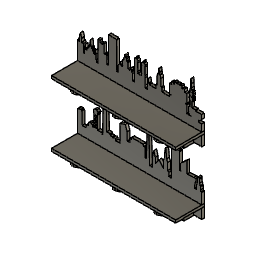
city-skyline-shelf (Autodesk Fusion 360 design; units mm, degrees)
Autodesk Fusion 360 part; units mm, degrees
(part 1 of 2)
sketch "Sketch1" plane through (0, 0, 0) normal (0, 1, 0) x (1, 0, 0) in component "tampere-background"
  line L0 (148.1857, -249.9146) -> (148.1857, -229.9217)
  line L1 (148.1857, -229.9217) -> (137.1896, -228.9221)
  line L2 (137.1896, -228.9221) -> (135.1904, -222.1945)
  line L3 (135.1904, -222.1945) -> (125.1939, -220.9248)
  line L4 (125.1939, -220.9248) -> (125.1939, -214.9267)
  line L5 (125.1939, -214.9267) -> (130.1924, -204.9302)
  line L6 (130.1924, -204.9302) -> (141.1885, -202.931)
  line L7 (141.1885, -202.931) -> (141.1885, -196.9329)
  line L8 (141.1885, -196.9329) -> (135.1904, -195.9333)
  line L9 (135.1904, -195.9333) -> (135.1904, -189.9352)
  line L10 (135.1904, -189.9352) -> (141.1885, -189.9352)
  line L11 (141.1885, -189.9352) -> (139.1893, -62.9787)
  spline S0 degree 3 poles (139.1893, -62.9787) (136.9773, -62.7994) (134.7652, -62.9787) (132.5486, -62.9787) knots 0 0 0 0 1 1 1 1
  line L12 (132.5486, -62.9787) -> (130.1919, -69.9764)
  line L13 (130.1919, -69.9764) -> (110.1989, -69.9764)
  line L14 (110.1989, -69.9764) -> (110.1989, -144.9508)
  line L15 (110.1989, -144.9508) -> (112.1981, -144.9508)
  line L16 (112.1981, -144.9508) -> (112.1981, -154.9473)
  line L17 (112.1981, -154.9473) -> (115.1974, -154.9473)
  line L18 (115.1974, -154.9473) -> (105.2004, -164.9438)
  line L19 (105.2004, -164.9438) -> (95.2039, -164.9438)
  line L20 (95.2039, -164.9438) -> (85.2075, -154.9473)
  line L21 (85.2075, -154.9473) -> (88.2062, -154.9473)
  line L22 (88.2062, -154.9473) -> (88.2062, -144.9508)
  line L23 (88.2062, -144.9508) -> (90.206, -144.9508)
  line L24 (90.206, -144.9508) -> (90.206, -73.9748)
  line L25 (90.206, -73.9748) -> (82.2087, -73.9748)
  line L26 (82.2087, -73.9748) -> (82.2087, -79.9729)
  line L27 (82.2087, -79.9729) -> (84.2079, -79.9729)
  line L28 (84.2079, -79.9729) -> (75.3474, -86.9706)
  line L29 (75.3474, -86.9706) -> (67.3501, -86.9706)
  line L30 (67.3501, -86.9706) -> (58.2168, -79.9729)
  line L31 (58.2168, -79.9729) -> (60.216, -79.9729)
  spline S1 degree 3 poles (60.216, -79.9729) (60.278, -75.6202) (60.3198, -71.3279) (60.216, -66.9771) knots 0 0 0 0 1 1 1 1
  line L32 (60.216, -66.9771) -> (50.2195, -66.9771)
  line L33 (50.2195, -66.9771) -> (45.221, -49.9829)
  line L34 (45.221, -49.9829) -> (25.2281, -49.9829)
  line L35 (25.2281, -49.9829) -> (25.2281, -119.9593)
  line L36 (25.2281, -119.9593) -> (18.2304, -119.9593)
  line L37 (18.2304, -119.9593) -> (18.2304, -124.1964)
  line L38 (18.2304, -124.1964) -> (7.2343, -124.1964)
  line L39 (7.2343, -124.1964) -> (7.2343, -119.9593)
  line L40 (7.2343, -119.9593) -> (0, -119.9593)
  line L41 (0, -119.9593) -> (0, 0)
  line L42 (0, 0) -> (345.1186, 0)
  line L43 (345.1186, 0) -> (690, 0)
  line L44 (690, 0) -> (690, -59.9799)
  line L45 (690, -59.9799) -> (684.0024, -59.9799)
  line L46 (684.0024, -59.9799) -> (684.0024, -69.9764)
  line L47 (684.0024, -69.9764) -> (682.8396, -84.9714)
  line L48 (682.8396, -84.9714) -> (681.0031, -87.9702)
  line L49 (681.0031, -87.9702) -> (678.0043, -98.9662)
  spline S2 degree 3 poles (678.0043, -98.9662) (677.0317, -105.2546) (676.0051, -113.2492) (676.0051, -116.2797) knots 0 0 0 0 1 1 1 1
  line L50 (676.0051, -116.2797) -> (676.0051, -122.2194)
  line L51 (676.0051, -122.2194) -> (672.0062, -128.2175)
  line L52 (672.0062, -128.2175) -> (667.855, -122.2194)
  line L53 (667.855, -122.2194) -> (667.8446, -116.2218)
  spline S3 degree 3 poles (667.8446, -116.2218) (667.8446, -110.2239) (667.0083, -102.9649) (666.0087, -98.9663) knots 0 0 0 0 1 1 1 1
  spline S4 degree 3 poles (666.0087, -98.9663) (665.5521, -97.1399) (664.009, -91.3596) (663.0094, -87.9702) knots 0 0 0 0 1 1 1 1
  line L54 (663.0094, -87.9702) -> (661.0102, -84.9714)
  line L55 (661.0102, -84.9714) -> (660.0044, -69.9764)
  line L56 (660.0044, -69.9764) -> (659.8473, -59.98)
  line L57 (659.8473, -59.98) -> (648.0149, -59.98)
  line L58 (648.0149, -59.98) -> (654.0022, -89.4967)
  spline S5 degree 2 poles (654.0022, -89.4967) (662.7338, -109.7693) (655.0121, -109.9624) knots 0 0 0 1 1 1
  line L59 (655.0121, -109.9624) -> (645.0156, -109.9624)
  line L60 (645.0156, -109.9624) -> (608.0285, -107.4615)
  line L61 (608.0285, -107.4615) -> (608.0285, -173.439)
  line L62 (608.0285, -173.439) -> (573.0405, -143.4491)
  line L63 (573.0405, -143.4491) -> (573.0405, -105.4623)
  line L64 (573.0405, -105.4623) -> (567.1684, -104.9644)
  line L65 (567.1684, -104.9644) -> (567.1684, -194.8345)
  line L66 (567.1684, -194.8345) -> (564.911, -196.7082)
  line L67 (564.911, -196.7082) -> (562.6535, -198.5813)
  line L68 (562.6535, -198.5813) -> (552.3032, -199.5303)
  line L69 (552.3032, -199.5303) -> (541.9528, -200.4788)
  line L70 (541.9528, -200.4788) -> (540.9429, -202.0977)
  line L71 (540.9429, -202.0977) -> (539.933, -203.7167)
  line L72 (539.933, -203.7167) -> (531.8355, -204.2168)
  line L73 (531.8355, -204.2168) -> (523.7385, -204.7168)
  line L74 (523.7385, -204.7168) -> (521.8984, -203.5494)
  line L75 (521.8984, -203.5494) -> (520.0584, -202.3824)
  line L76 (520.0584, -202.3824) -> (520.0584, -110.2563)
  line L77 (520.0584, -110.2563) -> (520.0584, -44.9849)
  line L78 (520.0584, -44.9849) -> (507.0631, -44.9849)
  line L79 (507.0631, -44.9849) -> (507.0631, -64.9779)
  line L80 (507.0631, -64.9779) -> (500.0654, -70.0678)
  line L81 (500.0654, -70.0678) -> (500.0654, -109.9623)
  spline S6 degree 3 poles (500.0654, -109.9623) (499.0397, -115.1717) (497.1361, -120.0402) (495.2121, -124.9573) knots 0 0 0 0 1 1 1 1
  line L82 (495.2121, -124.9573) -> (490.0689, -172.941)
  line L83 (490.0689, -172.941) -> (487.0701, -172.941)
  spline S7 degree 3 poles (487.0701, -172.941) (485.5899, -159.6869) (482.4701, -138.3214) (482.0716, -124.9573) knots 0 0 0 0 1 1 1 1
  spline S8 degree 3 poles (482.0716, -124.9573) (479.9709, -120.0963) (478.5362, -115.0454) (477.1124, -109.9623) knots 0 0 0 0 1 1 1 1
  line L84 (477.1124, -109.9623) -> (477.1124, -70.5457)
  line L85 (477.1124, -70.5457) -> (453.0818, -99.9658)
  line L86 (453.0818, -99.9658) -> (432.2829, -70.9873)
  line L87 (432.2829, -70.9873) -> (431.367, -99.9658)
  line L88 (431.367, -99.9658) -> (424.1157, -129.0399)
  line L89 (424.1157, -129.0399) -> (417.1263, -99.9658)
  spline S9 degree 3 poles (417.1263, -99.9658) (416.743, -92.2664) (416.0777, -52.6248) (415.0945, -44.9849) knots 0 0 0 0 1 1 1 1
  line L90 (415.0945, -44.9849) -> (401.0991, -44.9849)
  line L91 (401.0991, -44.9849) -> (396.1011, -189.9352)
  line L92 (396.1011, -189.9352) -> (386.1046, -189.9352)
  line L93 (386.1046, -189.9352) -> (381.1061, -69.9764)
  line L94 (381.1061, -69.9764) -> (375.108, -69.9764)
  line L95 (375.108, -69.9764) -> (375.108, -119.9593)
  line L96 (375.108, -119.9593) -> (367.0699, -119.9593)
  line L97 (367.0699, -119.9593) -> (364.1119, -129.9558)
  line L98 (364.1119, -129.9558) -> (301.1337, -129.9558)
  line L99 (301.1337, -129.9558) -> (298.1344, -119.9593)
  line L100 (298.1344, -119.9593) -> (290.1371, -119.9593)
  line L101 (290.1371, -119.9593) -> (290.1371, -99.9658)
  line L102 (290.1371, -99.9658) -> (275.1422, -99.9658)
  line L103 (275.1422, -99.9658) -> (275.1422, -144.9508)
  line L104 (275.1422, -144.9508) -> (265.1457, -174.9402)
  line L105 (265.1457, -174.9402) -> (235.1562, -164.9437)
  line L106 (235.1562, -164.9437) -> (235.398, -104.9643)
  line L107 (235.398, -104.9643) -> (235.1562, -69.9764)
  line L108 (235.1562, -69.9764) -> (210.1648, -69.9764)
  line L109 (210.1648, -69.9764) -> (210.1648, -80.0297)
  line L110 (210.1648, -80.0297) -> (198.1686, -79.9729)
  line L111 (198.1686, -79.9729) -> (198.1686, -76.9741)
  line L112 (198.1686, -76.9741) -> (192.171, -76.9741)
  line L113 (192.171, -76.9741) -> (192.171, -79.9729)
  line L114 (192.171, -79.9729) -> (180.1748, -80.0297)
  line L115 (180.1748, -80.0297) -> (180.1748, -87.9702)
  line L116 (180.1748, -87.9702) -> (161.479, -87.9702)
  line L117 (161.479, -87.9702) -> (159.1822, -189.9352)
  line L118 (159.1822, -189.9352) -> (165.1798, -189.9352)
  line L119 (165.1798, -189.9352) -> (165.1798, -195.9333)
  line L120 (165.1798, -195.9333) -> (159.1822, -196.9329)
  line L121 (159.1822, -196.9329) -> (159.1822, -202.931)
  line L122 (159.1822, -202.931) -> (170.1783, -204.9302)
  line L123 (170.1783, -204.9302) -> (175.1768, -214.9267)
  line L124 (175.1768, -214.9267) -> (175.1768, -220.9248)
  line L125 (175.1768, -220.9248) -> (165.1798, -222.4162)
  line L126 (165.1798, -222.4162) -> (163.1806, -228.9221)
  line L127 (163.1806, -228.9221) -> (152.1846, -229.9217)
  line L128 (152.1846, -229.9217) -> (152.1846, -249.9146)
  line L129 (152.1846, -249.9146) -> (148.1857, -249.9146)
  spline S10 degree 3 poles (100.203, -136.9959) (102.1721, -136.9959) (104.1414, -136.9018) (104.5464, -136.7143) knots 0 0 0 0 1 1 1 1
  spline S11 degree 3 poles (104.5464, -136.7143) (105.2015, -136.4111) (105.7342, -135.8601) (106.0094, -135.2012) knots 0 0 0 0 1 1 1 1
  spline S12 degree 3 poles (106.0094, -135.2012) (106.3456, -134.3964) (106.3078, -127.3549) (105.9634, -126.6109) knots 0 0 0 0 1 1 1 1
  spline S13 degree 3 poles (105.9634, -126.6109) (105.2904, -125.1573) (103.3727, -124.4944) (101.8736, -125.197) knots 0 0 0 0 1 1 1 1
  spline S14 degree 3 poles (101.8736, -125.197) (101.1385, -125.5415) (94.6738, -132.0446) (94.3945, -132.7206) knots 0 0 0 0 1 1 1 1
  spline S15 degree 3 poles (94.3945, -132.7206) (93.7727, -134.2253) (94.4455, -136.0597) (95.8595, -136.7143) knots 0 0 0 0 1 1 1 1
  spline S16 degree 3 poles (95.8595, -136.7143) (96.2645, -136.9018) (98.2339, -136.9959) (100.203, -136.9959) knots 0 0 0 0 1 1 1 1
  spline S17 degree 3 poles (97.3545, -120.9992) (97.7556, -120.9853) (98.1565, -120.8949) (98.5313, -120.7192) knots 0 0 0 0 1 1 1 1
  spline S18 degree 3 poles (98.5313, -120.7192) (99.2664, -120.3747) (105.7306, -113.8717) (106.0099, -113.1957) knots 0 0 0 0 1 1 1 1
  spline S19 degree 3 poles (106.0099, -113.1957) (106.6317, -111.6909) (105.9588, -109.8566) (104.5449, -109.2019) knots 0 0 0 0 1 1 1 1
  spline S20 degree 3 poles (104.5449, -109.2019) (103.7348, -108.8269) (96.6685, -108.8269) (95.8585, -109.2019) knots 0 0 0 0 1 1 1 1
  spline S21 degree 3 poles (95.8585, -109.2019) (95.2034, -109.5052) (94.6707, -110.0561) (94.3955, -110.715) knots 0 0 0 0 1 1 1 1
  spline S22 degree 3 poles (94.3955, -110.715) (94.0593, -111.5198) (94.097, -118.5614) (94.4415, -119.3053) knots 0 0 0 0 1 1 1 1
  spline S23 degree 3 poles (94.4415, -119.3053) (94.9462, -120.3955) (96.1511, -121.041) (97.3545, -120.9992) knots 0 0 0 0 1 1 1 1
  spline S24 degree 3 poles (100.203, -103.0075) (102.1721, -103.0075) (104.1414, -102.9135) (104.5464, -102.726) knots 0 0 0 0 1 1 1 1
  spline S25 degree 3 poles (104.5464, -102.726) (105.2015, -102.4227) (105.7342, -101.8718) (106.0094, -101.2129) knots 0 0 0 0 1 1 1 1
  spline S26 degree 3 poles (106.0094, -101.2129) (106.3456, -100.4081) (106.3078, -93.3665) (105.9634, -92.6226) knots 0 0 0 0 1 1 1 1
  spline S27 degree 3 poles (105.9634, -92.6226) (105.2904, -91.1689) (103.3727, -90.5061) (101.8736, -91.2087) knots 0 0 0 0 1 1 1 1
  spline S28 degree 3 poles (101.8736, -91.2087) (101.1385, -91.5532) (94.6738, -98.0562) (94.3945, -98.7322) knots 0 0 0 0 1 1 1 1
  spline S29 degree 3 poles (94.3945, -98.7322) (93.7727, -100.237) (94.4455, -102.0713) (95.8595, -102.726) knots 0 0 0 0 1 1 1 1
  spline S30 degree 3 poles (95.8595, -102.726) (96.2645, -102.9135) (98.2339, -103.0075) (100.203, -103.0075) knots 0 0 0 0 1 1 1 1
  spline S31 degree 3 poles (97.3545, -87.0109) (97.7556, -86.997) (98.1565, -86.9065) (98.5313, -86.7309) knots 0 0 0 0 1 1 1 1
  spline S32 degree 3 poles (98.5313, -86.7309) (99.2664, -86.3863) (105.7306, -79.8833) (106.0099, -79.2073) knots 0 0 0 0 1 1 1 1
  spline S33 degree 3 poles (106.0099, -79.2073) (106.6317, -77.7025) (105.9588, -75.8682) (104.5449, -75.2136) knots 0 0 0 0 1 1 1 1
  spline S34 degree 3 poles (104.5449, -75.2136) (103.7348, -74.8385) (96.6685, -74.8385) (95.8585, -75.2136) knots 0 0 0 0 1 1 1 1
  spline S35 degree 3 poles (95.8585, -75.2136) (95.2034, -75.5168) (94.6707, -76.0678) (94.3955, -76.7266) knots 0 0 0 0 1 1 1 1
  spline S36 degree 3 poles (94.3955, -76.7266) (94.0593, -77.5314) (94.097, -84.573) (94.4415, -85.317) knots 0 0 0 0 1 1 1 1
  spline S37 degree 3 poles (94.4415, -85.317) (94.9462, -86.4072) (96.1511, -87.0526) (97.3545, -87.0109) knots 0 0 0 0 1 1 1 1
  line L130 (138, 0) -> (276, 0)
  line L131 (414, 0) -> (552, 0)
  line L132 (0, 0) -> (690, 0)
  line L133 (690, 70) -> (0, 70)
  line L134 (138, 15.1) -> (138, 0)
  line L135 (0, 15.1) -> (0, 70)
  line L136 (276, 0) -> (414, 0)
  line L137 (414, 0) -> (414, 15.1)
  line L138 (276, 15.1) -> (276, 0)
  line L139 (552, 0) -> (552, 15.1)
  line L140 (690, 15.1) -> (690, 70)
  line L141 (337.45, 15.1) -> (337.45, 44.6036)
  line L142 (337.45, 44.6036) -> (352.55, 44.6036)
  line L143 (352.55, 44.6036) -> (352.55, 15.1)
  line L144 (106, 15.1) -> (106, 44.6036)
  line L145 (106, 44.6036) -> (121.1, 44.6036)
  line L146 (121.1, 44.6036) -> (121.1, 15.1)
  line L147 (584, 15.1) -> (584, 44.6036)
  line L148 (584, 44.6036) -> (568.9, 44.6036)
  line L149 (568.9, 44.6036) -> (568.9, 15.1)
  line L150 (121.1, 15.1) -> (138, 15.1)
  line L151 (106, 15.1) -> (0, 15.1)
  line L152 (276, 15.1) -> (337.45, 15.1)
  line L153 (352.55, 15.1) -> (414, 15.1)
  line L154 (552, 15.1) -> (568.9, 15.1)
  line L155 (584, 15.1) -> (690, 15.1)
  dimension "d110" = 70
  dimension "d112" = 15.1
  dimension "d113" = 138
  dimension "d115" = 138
  dimension "d116" = 15.1
  dimension "d117" = 138
  dimension "d118" = 15.1
  dimension "d119" = 138
  dimension "d127" = 15.1
  dimension "d128" = 61.45
  dimension "d129" = 29.5036
  dimension "d130" = 106
  dimension "d131" = 15.1
  dimension "d132" = 29.5036
  dimension "d133" = 106
  dimension "d134" = 29.5036
  dimension "d135" = 15.1
  dimension "d158" = 15.1
  dimension "d159" = 15.1
  dimension "d160" = 15.1
  constraint horizontal L130
  constraint coincident L42 L130.start
  constraint horizontal L131
  constraint coincident L43 L131.start
  constraint horizontal L132
  constraint horizontal L133
  constraint coincident L41.end L42.start
  constraint perpendicular L132 L134
  constraint perpendicular L133 L135
  constraint equal L132 L133
  constraint horizontal L136
  constraint vertical L137
  constraint vertical L138
  constraint coincident L132 L130.end
  constraint coincident L43 L131.end
  constraint perpendicular L43 L139
  constraint perpendicular L133 L140
  constraint vertical L141
  constraint horizontal L142
  constraint vertical L143
  constraint vertical L144
  constraint horizontal L145
  constraint vertical L146
  constraint vertical L147
  constraint horizontal L148
  constraint vertical L149
  constraint horizontal L151
  constraint horizontal L150
  constraint perpendicular L141 L152
  constraint perpendicular L137 L153
  constraint perpendicular L149 L154
  constraint perpendicular L140 L155
  constraint collinear L44 L140
  constraint collinear L41 L135
  measures "d110" distance of L43.end L133.start
  measures "d112" distance of L130.start L134.start
  measures "d113" distance of L134.start L135.start
  measures "d115" distance of L137.end L138.start
  measures "d116" distance of L131.start L137.end
  measures "d117" distance of L134 L138
  measures "d118" distance of L131.end L139.end
  measures "d119" distance of L139.end L140.start
  measures "d127" distance of L141.end L142.end
  measures "d128" distance of L137.end L143
  measures "d129" distance of L141.start L141.end
  measures "d130" distance of L135 L144
  measures "d131" distance of L144.end L145.end
  measures "d132" distance of L146.end L145.end
  measures "d133" distance of L140 L147
  measures "d134" distance of L149.end L148.end
  measures "d135" distance of L147.end L148.end
  measures "d158" distance of L42 L151
  measures "d159" distance of L132 L155
  measures "d160" distance of L42 L152
extrude "Extrude1" add sketch "Sketch1" along normal blind 15 contours L0 L1 L2 L3 L4 L5 L6 L7 L8 L9 L10 L11 S0 L12 L13 L14 L15 L16 L17 L18 L19 L20 L21 L22 L23 L24 L25 L26 L27 L28 L29 L30 L31 S1 L32 L33 L34 L35 L36 L37 L38 L39 L40 L41 L42 L43 L44 L45 L46 L47 L48 L49 S2 L50 L51 L52 L53 S3 S4 L54 L55 L56 L57 L58 S5 L59 L60 L61 L62 L63 L64 L65 L66 L67 L68 L69 L70 L71 L72 L73 L74 L75 L76 L77 L78 L79 L80 L81 S6 L82 L83 S7 S8 L84 L85 L86 L87 L88 L89 S9 L90 L91 L92 L93 L94 L95 L96 L97 L98 L99 L100 L101 L102 L103 L104 L105 L106 L107 L108 L109 L110 L111 L112 L113 L114 L115 L116 L117 L118 L119 L120 L121 L122 L123 L124 L125 L126 L127 L128 L129 L130 L131 L132 L136 | L42 L43 L130 L131 L132 L133 L134 L135 L137 L138 L139 L140 L141 L142 L143 L144 L145 L146 L147 L148 L149 L150 L151 L152 L153 L154 L155 makes body 1 in component "tampere-background"
sketch "Sketch2" plane through (0, 0, 0) normal (0, 0, 1) x (1, 0, 0) in component "shelf"
  line L0 (0, 0) -> (690, 0)
  line L1 (690, 0) -> (690, -145)
  line L2 (690, -145) -> (0, -145)
  line L3 (0, -145) -> (0, 0)
  line L4 (0, 0) -> (138, 0)
  line L5 (138, 0) -> (138, 15)
  line L6 (138, 15) -> (0, 15)
  line L7 (0, 15) -> (0, 0)
  line L8 (552, 0) -> (690, 0)
  line L9 (690, 0) -> (690, 15)
  line L10 (690, 15) -> (552, 15)
  line L11 (552, 15) -> (552, 0)
  line L12 (276, 0) -> (414, 0)
  line L13 (414, 0) -> (414, 15)
  line L14 (414, 15) -> (276, 15)
  line L15 (276, 15) -> (276, 0)
  dimension "d12" = 690
  dimension "d13" = 145
  dimension "d14" = 138
  dimension "d16" = 15
  dimension "d17" = 138
  dimension "d18" = 15
  dimension "d30" = 138
  dimension "d31" = 15
  dimension "d32" = 138
  constraint horizontal L0
  constraint vertical L1
  constraint horizontal L2
  constraint vertical L3
  constraint coincident L0.start L3.end
  constraint horizontal L4
  constraint vertical L5
  constraint horizontal L6
  constraint vertical L7
  constraint coincident L0 L3.end
  constraint horizontal L8
  constraint vertical L9
  constraint horizontal L10
  constraint vertical L11
  constraint coincident L0 L8.start
  constraint coincident L0.start L7
  constraint coincident L0.end L9
  constraint horizontal L12
  constraint vertical L13
  constraint horizontal L14
  constraint vertical L15
  constraint coincident L0 L12.start
  measures "d12" distance of L1.end L2.end
  measures "d13" distance of L0.start L2.end
  measures "d14" distance of L5.end L6.end
  measures "d16" distance of L0.start L6.end
  measures "d17" distance of L9.end L10.end
  measures "d18" distance of L0.end L9.end
  measures "d30" distance of L13.end L14.end
  measures "d31" distance of L12.end L13.end
  measures "d32" distance of L11 L13
extrude "Extrude1'" add sketch "Sketch2" along normal blind 15 separate body makes body 2 in component "shelf"
move_body "Move1" bodies 2 to x (1, 0, 0) y (0, 1, 0) z (0, 0, 1) at (0, 0, -75) in component "shelf"
sketch "Sketch4" plane through (0, 0, -75) normal (0, 0, -1) x (1, 0, 0)
  line L0 (414, -15) -> (414, 0)
  line L1 (414, 0) -> (552, 0)
  line L2 (552, 0) -> (552, -15)
  line L3 (552, -15) -> (690, -15)
  line L4 (690, -15) -> (690, 145)
  line L5 (690, 145) -> (0, 145)
  line L6 (0, 145) -> (0, -15)
  line L7 (0, -15) -> (138, -15)
  line L8 (138, -15) -> (138, 0)
  line L9 (138, 0) -> (276, 0)
  line L10 (276, 0) -> (276, -15)
  line L11 (276, -15) -> (414, -15)
  line L12 (106, -15) -> (121.1, -15)
  line L13 (121.1, -15) -> (121.1, 141.8)
  line L14 (121.1, 141.8) -> (106, 141.8)
  line L15 (106, 141.8) -> (106, -15)
  line L16 (337.45, -15) -> (352.55, -15)
  line L17 (352.55, -15) -> (352.55, 141.8)
  line L18 (352.55, 141.8) -> (337.45, 141.8)
  line L19 (337.45, 141.8) -> (337.45, -15)
  line L20 (568.9, -15) -> (584, -15)
  line L21 (584, -15) -> (584, 141.8)
  line L22 (584, 141.8) -> (568.9, 141.8)
  line L23 (568.9, 141.8) -> (568.9, -15)
  line L24 (121.1, 113.6693) -> (337.45, 113.6693) construction
  line L25 (352.55, 113.6693) -> (568.9, 113.6693) construction
  line L26 (0, 99.2167) -> (690, 99.2167)
  line L27 (690, 99.2167) -> (690, 45.7833)
  line L28 (690, 45.7833) -> (0, 45.7833)
  line L29 (0, 45.7833) -> (0, 99.2167)
  line L30 (690, 72.5) -> (690, 65) construction
  dimension "d43" = 15.1
  dimension "d44" = 156.8
  dimension "d45" = 106
  dimension "d46" = 106
  dimension "d48" = 53.4333
  dimension "d145" = 45.7833
  constraint horizontal L12
  constraint vertical L13
  constraint horizontal L14
  constraint vertical L15
  constraint horizontal L16
  constraint vertical L17
  constraint horizontal L18
  constraint vertical L19
  constraint horizontal L20
  constraint vertical L21
  constraint horizontal L22
  constraint vertical L23
  constraint equal L14 L18
  constraint equal L18 L22
  constraint equal L13 L17
  constraint equal L17 L21
  constraint coincident L13 L24.start
  constraint coincident L19 L24.end
  constraint perpendicular L19 L24
  constraint coincident L17 L25.start
  constraint coincident L23 L25.end
  constraint perpendicular L23 L25
  constraint equal L24 L25
  constraint horizontal L26
  constraint vertical L27
  constraint horizontal L28
  constraint vertical L29
  constraint midpoint L27 L30.start
  constraint midpoint L4 L30.end
  constraint coincident L19 L16.start
  constraint coincident L20.start L23.end
  constraint coincident L12.start L15.end
  constraint coincident L16.start L19.end
  constraint collinear L11 L16
  constraint collinear L3 L20
  constraint collinear L7 L12
  constraint collinear L6 L29
  constraint collinear L4 L27
  measures "d43" distance of L17.end L18.end
  measures "d44" distance of L16.end L17.end
  measures "d45" distance of origin L15
  measures "d46" distance of L3.end L21
  measures "d48" distance of L26.end L27.end
  measures "d145" distance of L1 L28
extrude "Extrude2" cut sketch "Sketch4" against normal blind 1.875 contours L11 L16 L17 L19 L28 | L17 L19 L26 L28 | L17 L23 L26 L28 | L13 L19 L26 L28 | L17 L18 L19 L26 | L3 L20 L21 L23 L28 | L21 L23 L26 L28 | L13 L15 L26 L28 | L7 L12 L13 L15 L28 | L21 L22 L23 L26 | L4 L21 L26 L27 L28 | L13 L14 L15 L26 | L6 L15 L26 L28 L29 bodies 2 in component "shelf"
sketch "Sketch1 (2)" plane through (0, 0, 0) normal (0, 0, 1) x (1, 0, 0) in component "support-bar"
sketch "Sketch2 (2)" plane through (0, 0, 0) normal (0, 0, 1) x (1, 0, 0) in component "support-bar"
  line L0 (0, 0) -> (690, 0)
  line L1 (690, 0) -> (690, -53.3333)
  line L2 (690, -53.3333) -> (0, -53.3333)
  line L3 (0, -53.3333) -> (0, 0)
  dimension "d52" = 690
  dimension "d53" = 53.3333
  constraint horizontal L0
  constraint vertical L1
  constraint horizontal L2
  constraint vertical L3
  constraint coincident L0.start L3.end
  measures "d52" distance of L0.start L0.end
  measures "d53" distance of L0.start L2.end
extrude "Extrude1''" add sketch "Sketch2 (2)" along normal blind 15 separate body makes body 3 in component "support-bar"
move_body "Move1'" bodies 3 to x (1, 0, 0) y (0, 1, 0) z (0, 0, 1) at (0, 0, -90) in component "support-bar"
sketch "Sketch1 (3)" plane through (0, 0, 0) normal (1, 0, 0) x (0, 1, 0) in component "triangle-support"
  line L0 (-15, 0) -> (-150, 0)
  line L1 (-155.4076, -18.4118) -> (-15.4076, -108.4118)
  line L2 (0, -100) -> (0, -56.925)
  arc A0 (-15.4076, -108.4118) -> (0, -100) centre (-10, -100) ccw
  arc A1 (-150, 0) -> (-155.4076, -18.4118) centre (-150, -10) ccw
  line L3 (0, 0) -> (0, -110) construction
  line L4 (0, 0) -> (-160, 0) construction
  line L5 (0, -110) -> (-35, -110) construction
  line L6 (-160, 0) -> (-160, -24.9001) construction
  line L7 (-45, -31.3786) -> (-77.5293, -31.3786)
  line L8 (-80.2331, -40.5845) -> (-47.7038, -61.4962)
  line L9 (-40, -57.2903) -> (-40, -36.3786)
  arc A2 (-47.7038, -61.4962) -> (-40, -57.2903) centre (-45, -57.2903) ccw
  arc A3 (-40, -36.3786) -> (-45, -31.3786) centre (-45, -36.3786) ccw
  arc A4 (-77.5293, -31.3786) -> (-80.2331, -40.5845) centre (-77.5293, -36.3786) ccw
  line L10 (-60.7833, 0) -> (-114.2167, 0)
  line L11 (-114.2167, 0) -> (-114.2167, -15)
  line L12 (-114.2167, -15) -> (-60.7833, -15)
  line L13 (-60.7833, -15) -> (-60.7833, 0)
  line L14 (0, -56.925) -> (-15, -56.925)
  line L15 (-15, -56.925) -> (-15, 0)
  line L16 (-15, 0) -> (0, 0)
  line L17 (0, 0) -> (0, -31.3786)
  line L18 (0, -31.3786) -> (-15, -31.3786)
  line L19 (-66.4844, -49.4229) -> (-78.3811, -67.9288) construction
  dimension "d60" = 10
  dimension "d63" = 110
  dimension "d64" = 160
  dimension "d65" = 5
  dimension "d66" = 5
  dimension "d67" = 40
  dimension "d68" = 31.3786
  dimension "d71" = 53.4333
  dimension "d72" = 15
  dimension "d124" = 15
  dimension "d125" = 56.925
  dimension "d126" = 15
  dimension "d136" = 45.7833
  dimension "d186" = 22
  constraint horizontal L0
  constraint perpendicular L0 L2
  constraint tangent L2 A0
  constraint tangent L1 A0
  constraint tangent L1 A1
  constraint tangent L0 A1
  constraint equal A0 A1
  constraint coincident L3.start L4.start
  constraint perpendicular L0 L3
  constraint collinear L2 L3
  constraint perpendicular L3 L4
  constraint collinear L0 L4
  constraint horizontal L5
  constraint tangent A0 L5
  constraint coincident L3.end L5.start
  constraint vertical L6
  constraint tangent A1 L6
  constraint coincident L4.end L6.start
  constraint parallel L4 L7
  constraint perpendicular L7 L9
  constraint tangent L8 A2
  constraint tangent L9 A2
  constraint tangent L9 A3
  constraint tangent L7 A3
  constraint equal A2 A3
  constraint tangent L7 A4
  constraint tangent L8 A4
  constraint horizontal L10
  constraint vertical L11
  constraint horizontal L12
  constraint vertical L13
  constraint coincident L4 L10.start
  constraint coincident L0 L10.start
  constraint horizontal L14
  constraint vertical L15
  constraint coincident L2 L14.start
  constraint coincident L3 L2.end
  constraint coincident L4 L0.start
  constraint coincident L2.end L14.start
  constraint coincident L0.start L15.end
  constraint horizontal L16
  constraint vertical L17
  constraint horizontal L18
  constraint collinear L7 L18
  constraint parallel L1 L8
  constraint coincident L8 L19.start
  constraint coincident L1 L19.end
  constraint perpendicular L1 L19
  constraint coincident L15 L18.end
  measures "d60" radius of A0
  measures "d63" distance of L3.start L3.end
  measures "d64" distance of L3.start L4.end
  measures "d65" radius of A2
  measures "d66" radius of A4
  measures "d67" distance of L2 L9
  measures "d68" distance of L0 L7
  measures "d71" distance of L11.end L12.end
  measures "d72" distance of L10.end L11.end
  measures "d124" distance of L2.end L14.end
  measures "d125" distance of L0.start L14.end
  measures "d126" distance of L0.start L3.start
  measures "d136" distance of L13 L15
  measures "d186" distance of L19.start L19.end
extrude "Extrude1'''" add sketch "Sketch1 (3)" along normal blind 15 separate body contours L0 L1 L2 A0 A1 L11 L12 L13 L14 L15 | L15 L16 L17 L18 makes body 4 in component "triangle-support"
move_body "Move1''" bodies 4 to x (1, 0, 0) y (0, 1, 0) z (0, 0, 1) at (0, 0, -50) in component "triangle-support"
sketch "Sketch1 (4)" plane through (0, 0, 0) normal (0, 1, 0) x (1, 0, 0) in component "munich-background"
  line L0 (629, -226.9948) -> (628, -204.9948)
  line L1 (628, -204.9948) -> (627, -184.9948)
  line L2 (627, -184.9948) -> (625, -174.9948)
  line L3 (625, -174.9948) -> (625, -169.9948)
  line L4 (625, -169.9948) -> (623, -169.9948)
  spline S0 degree 3 poles (623, -169.9948) (622.0426, -169.9666) (621, -168.9522) (621, -167.9948) knots 0 0 0 0 1 1 1 1
  spline S1 degree 3 poles (621, -167.9948) (621.0282, -166.9529) (622.0426, -166.0229) (623, -165.9948) knots 0 0 0 0 1 1 1 1
  line L5 (623, -165.9948) -> (625, -165.9948)
  line L6 (625, -165.9948) -> (625, -159.9948)
  line L7 (625, -159.9948) -> (619, -157.9948)
  line L8 (619, -157.9948) -> (619, -147.9948)
  line L9 (619, -147.9948) -> (625, -145.9948)
  line L10 (625, -145.9948) -> (625, -139.9948)
  line L11 (625, -139.9948) -> (619, -139.9948)
  line L12 (619, -139.9948) -> (619, -137.9948)
  spline S2 degree 2 poles (619, -137.9948) (621, -137.9948) (621, -134.9948) knots 0 0 0 1 1 1
  spline S3 degree 2 poles (621, -134.9948) (621, -131.9948) (619, -131.9948) knots 0 0 0 1 1 1
  line L13 (619, -131.9948) -> (619, -129.9948)
  spline S4 degree 2 poles (619, -129.9948) (621, -129.9948) (621, -126.9948) knots 0 0 0 1 1 1
  spline S5 degree 2 poles (621, -126.9948) (621, -123.9948) (619, -123.9948) knots 0 0 0 1 1 1
  line L14 (619, -123.9948) -> (619, -121.9948)
  line L15 (619, -121.9948) -> (625, -121.9948)
  line L16 (625, -121.9948) -> (624, -89.9948)
  line L17 (624, -89.9948) -> (617, -89.9948)
  line L18 (617, -89.9948) -> (617, -61.9948)
  spline S6 degree 3 poles (617, -61.9948) (617, -55.9948) (623, -47.9948) (630, -47.9948) knots 0 0 0 0 1 1 1 1
  line L19 (630, -47.9948) -> (607.0867, -47.9948)
  line L20 (607.0867, -47.9948) -> (607.0867, -89.9948)
  line L21 (607.0867, -89.9948) -> (599, -93.9948)
  line L22 (599, -93.9948) -> (607.1813, -97.9948)
  line L23 (607.1813, -97.9948) -> (607, -144.9948)
  line L24 (607, -144.9948) -> (595, -144.9948)
  line L25 (595, -144.9948) -> (594.9041, -159.9948)
  line L26 (594.9041, -159.9948) -> (587, -159.9948)
  spline S7 degree 2 poles (587, -159.9948) (587, -153.0676) (580, -154.9948) knots 0 0 0 1 1 1
  line L27 (580, -154.9948) -> (580, -166.9948)
  line L28 (580, -166.9948) -> (570, -166.9948)
  line L29 (570, -166.9948) -> (570, -164.9948)
  line L30 (570, -164.9948) -> (564, -164.9948)
  line L31 (564, -164.9948) -> (564, -166.9948)
  line L32 (564, -166.9948) -> (553, -166.9948)
  line L33 (553, -166.9948) -> (553, -164.9948)
  line L34 (553, -164.9948) -> (547, -164.9948)
  line L35 (547, -164.9948) -> (547, -166.9948)
  line L36 (547, -166.9948) -> (537, -166.9948)
  line L37 (537, -166.9948) -> (537, -154.9948)
  spline S8 degree 2 poles (537, -154.9948) (529.9203, -153.1452) (530, -159.9948) knots 0 0 0 1 1 1
  line L38 (530, -159.9948) -> (522, -159.9948)
  line L39 (522, -159.9948) -> (521.991, -145.2144)
  line L40 (521.991, -145.2144) -> (510, -145.2144)
  line L41 (510, -145.2144) -> (510, -97.9948)
  line L42 (510, -97.9948) -> (518, -93.9948)
  line L43 (518, -93.9948) -> (510, -89.9948)
  line L44 (510, -89.9948) -> (510, -82.9948)
  line L45 (510, -82.9948) -> (469, -82.9948)
  line L46 (469, -82.9948) -> (469, -102.9948)
  line L47 (469, -102.9948) -> (463, -102.9948)
  line L48 (463, -102.9948) -> (463, -144.9948)
  line L49 (463, -144.9948) -> (459, -159.9948)
  line L50 (459, -159.9948) -> (456, -159.9948)
  line L51 (456, -159.9948) -> (456, -169.9948)
  line L52 (456, -169.9948) -> (454, -169.9948)
  line L53 (454, -169.9948) -> (453, -187.9948)
  spline S9 degree 2 poles (453, -187.9948) (452.115, -192.5346) (451, -187.9948) knots 0 0 0 1 1 1
  line L54 (451, -187.9948) -> (450, -169.9948)
  line L55 (450, -169.9948) -> (448, -169.9948)
  line L56 (448, -169.9948) -> (448, -159.9948)
  line L57 (448, -159.9948) -> (445, -159.9948)
  line L58 (445, -159.9948) -> (441, -144.9948)
  line L59 (441, -144.9948) -> (441, -102.9948)
  line L60 (441, -102.9948) -> (435, -102.9948)
  line L61 (435, -102.9948) -> (435, -82.9948)
  line L62 (435, -82.9948) -> (398, -82.9948)
  line L63 (398, -82.9948) -> (398, -85.9948)
  spline S10 degree 2 poles (398, -85.9948) (396, -86.1933) (396, -89.9948) knots 0 0 0 1 1 1
  line L64 (396, -89.9948) -> (395, -89.9948)
  line L65 (395, -89.9948) -> (393, -109.9948)
  spline S11 degree 2 poles (393, -109.9948) (392.5376, -112.3045) (392, -109.9948) knots 0 0 0 1 1 1
  line L66 (392, -109.9948) -> (390, -89.9948)
  line L67 (390, -89.9948) -> (389, -89.9948)
  spline S12 degree 2 poles (389, -89.9948) (388.9155, -85.9399) (387, -85.9948) knots 0 0 0 1 1 1
  line L68 (387, -85.9948) -> (387, -77.9948)
  line L69 (387, -77.9948) -> (386, -77.9948)
  spline S13 degree 2 poles (386, -77.9948) (385, -77.9804) (385, -76.9948) knots 0 0 0 1 1 1
  line L70 (385, -76.9948) -> (385, -74.9948)
  spline S14 degree 2 poles (385, -74.9948) (385.0563, -73.9529) (385.9771, -73.9948) knots 0 0 0 1 1 1
  line L71 (385.9771, -73.9948) -> (387, -73.9948)
  line L72 (387, -73.9948) -> (387, -66.9948)
  line L73 (387, -66.9948) -> (386, -66.9948)
  spline S15 degree 2 poles (386, -66.9948) (385.0282, -66.9804) (385, -65.9948) knots 0 0 0 1 1 1
  line L74 (385, -65.9948) -> (385, -62.9948)
  spline S16 degree 2 poles (385, -62.9948) (385.0282, -62.0092) (385.9208, -61.9948) knots 0 0 0 1 1 1
  line L75 (385.9208, -61.9948) -> (387, -61.9948)
  line L76 (387, -61.9948) -> (387, -55.0799)
  line L77 (387, -55.0799) -> (374.9999, -54.9948)
  line L78 (374.9999, -54.9948) -> (375, -104.9947)
  line L79 (375, -104.9947) -> (375, -114.9948)
  line L80 (375, -114.9948) -> (374, -154.9948)
  line L81 (374, -154.9948) -> (374.9999, -164.8056)
  spline S17 degree 2 poles (374.9999, -164.8056) (375.0125, -172.3049) (370.0002, -172.4175) knots 0 0 0 1 1 1
  line L82 (370.0002, -172.4175) -> (366, -172.9952)
  line L83 (366, -172.9952) -> (365.2558, -179.9948)
  spline S18 degree 2 poles (365.2558, -179.9948) (365.1621, -180.2093) (365.0315, -180.2361) knots 0 0 0 1 1 1
  spline S19 degree 3 poles (365.0315, -180.2361) (364.9532, -180.2522) (364.8619, -180.2007) (364.7696, -179.9948) knots 0 0 0 0 1 1 1 1
  line L84 (364.7696, -179.9948) -> (364.0001, -172.9952)
  line L85 (364.0001, -172.9952) -> (360.0003, -172.4454)
  spline S20 degree 2 poles (360.0003, -172.4454) (354.988, -172.4454) (355.0001, -164.9952) knots 0 0 0 1 1 1
  spline S21 degree 3 poles (355.0001, -164.9952) (354.9567, -160.9839) (356.0148, -158.9586) (356.0001, -154.9948) knots 0 0 0 0 1 1 1 1
  spline S22 degree 3 poles (356.0001, -154.9948) (355.9538, -142.5116) (355.0924, -127.2661) (355, -114.9948) knots 0 0 0 0 1 1 1 1
  spline S23 degree 3 poles (355, -114.9948) (354.9666, -109.6615) (355, -110.328) (355, -104.9947) knots 0 0 0 0 1 1 1 1
  line L86 (355, -104.9947) -> (335.0002, -104.9947)
  line L87 (335.0002, -104.9947) -> (335.0002, -114.9946)
  line L88 (335.0002, -114.9946) -> (333.9998, -154.9947)
  line L89 (333.9998, -154.9947) -> (335.0002, -164.8055)
  spline S24 degree 2 poles (335.0002, -164.8055) (335.0123, -172.3048) (330, -172.4174) knots 0 0 0 1 1 1
  line L90 (330, -172.4174) -> (326.0002, -172.9946)
  line L91 (326.0002, -172.9946) -> (325.2561, -179.9947)
  spline S25 degree 2 poles (325.2561, -179.9947) (325.0157, -180.5438) (324.7693, -179.9947) knots 0 0 0 1 1 1
  line L92 (324.7693, -179.9947) -> (323.9998, -172.9946)
  line L93 (323.9998, -172.9946) -> (320.0001, -172.4453)
  spline S26 degree 2 poles (320.0001, -172.4453) (314.9878, -172.4453) (314.9999, -164.9946) knots 0 0 0 1 1 1
  spline S27 degree 3 poles (314.9999, -164.9946) (314.9565, -160.9833) (316.0145, -158.9586) (315.9998, -154.9947) knots 0 0 0 0 1 1 1 1
  spline S28 degree 3 poles (315.9998, -154.9947) (315.9497, -141.4944) (314.9542, -128.2723) (314.9999, -114.9946) knots 0 0 0 0 1 1 1 1
  spline S29 degree 3 poles (314.9999, -114.9946) (315.068, -95.1907) (315.077, -75.3722) (314.9999, -54.9946) knots 0 0 0 0 1 1 1 1
  line L94 (314.9999, -54.9946) -> (305, -54.9946)
  line L95 (305, -54.9946) -> (305, -89.9945)
  spline S30 degree 3 poles (305, -89.9945) (303.7059, -91.7055) (304.9998, -92.995) (299.9476, -95.003) knots 0 0 0 0 1 1 1 1
  line L96 (299.9476, -95.003) -> (299.9998, -94.995)
  spline S31 degree 2 poles (299.9998, -94.995) (301.2741, -97.4864) (299.9998, -99.9952) knots 0 0 0 1 1 1
  spline S32 degree 2 poles (299.9998, -99.9952) (298.9999, -100.9952) (296.9999, -100.9952) knots 0 0 0 1 1 1
  spline S33 degree 3 poles (296.9999, -100.9952) (296.5852, -100.9952) (295.9435, -108.302) (294.9995, -109.9952) knots 0 0 0 0 1 1 1 1
  spline S34 degree 3 poles (294.9995, -109.9952) (294.3124, -111.2275) (293.6213, -111.1943) (292.9997, -109.9952) knots 0 0 0 0 1 1 1 1
  spline S35 degree 3 poles (292.9997, -109.9952) (292.7185, -109.4528) (291.5277, -101.0168) (290.9998, -100.9952) knots 0 0 0 0 1 1 1 1
  spline S36 degree 2 poles (290.9998, -100.9952) (288.448, -100.891) (288, -99.9952) knots 0 0 0 1 1 1
  spline S37 degree 3 poles (288, -99.9952) (287.104, -98.2441) (287.9639, -95.2685) (288, -94.995) knots 0 0 0 0 1 1 1 1
  spline S38 degree 3 poles (288, -94.995) (287, -94.995) (280, -94.9951) (279.9999, -99.9952) knots 0 0 0 0 1 1 1 1
  line L97 (279.9999, -99.9952) -> (279.9999, -129.9947)
  line L98 (279.9999, -129.9947) -> (274.9997, -130.0345)
  spline S39 degree 2 poles (274.9997, -130.0345) (273.0484, -130.0345) (272.9998, -134.9949) knots 0 0 0 1 1 1
  line L99 (272.9998, -134.9949) -> (272.9998, -144.9948)
  spline S40 degree 2 poles (272.9998, -144.9948) (270.9569, -147.9665) (268.0001, -147.9946) knots 0 0 0 1 1 1
  line L100 (268.0001, -147.9946) -> (268.0001, -158.995)
  spline S41 degree 3 poles (268.0001, -158.995) (264.6368, -165.7639) (265.3042, -165.5588) (262, -158.995) knots 0 0 0 0 1 1 1 1
  line L101 (262, -158.995) -> (262, -147.9946)
  spline S42 degree 2 poles (262, -147.9946) (259.0151, -147.9664) (256.9998, -144.9948) knots 0 0 0 1 1 1
  line L102 (256.9998, -144.9948) -> (256.9998, -134.9949)
  spline S43 degree 2 poles (256.9998, -134.9949) (257.0309, -129.9947) (254.9999, -129.9947) knots 0 0 0 1 1 1
  line L103 (254.9999, -129.9947) -> (250.0002, -129.9947)
  spline S44 degree 3 poles (250.0002, -129.9947) (249.9942, -127.4904) (250.0002, -111.087) (250.0002, -99.995) knots 0 0 0 0 1 1 1 1
  spline S45 degree 3 poles (250.0002, -99.995) (250.0002, -94.995) (243.0002, -94.9948) (242.0002, -94.9948) knots 0 0 0 0 1 1 1 1
  spline S46 degree 2 poles (242.0002, -94.9948) (243.2745, -97.4861) (242.0002, -99.995) knots 0 0 0 1 1 1
  spline S47 degree 2 poles (242.0002, -99.995) (240.9999, -100.9949) (238.9999, -100.9949) knots 0 0 0 1 1 1
  spline S48 degree 3 poles (238.9999, -100.9949) (238.5851, -100.9949) (237.944, -108.3017) (237, -109.9949) knots 0 0 0 0 1 1 1 1
  spline S49 degree 3 poles (237, -109.9949) (236.3129, -111.2273) (235.6218, -111.194) (235.0001, -109.9949) knots 0 0 0 0 1 1 1 1
  spline S50 degree 3 poles (235.0001, -109.9949) (234.7189, -109.4525) (233.5282, -101.0165) (233.0002, -100.9949) knots 0 0 0 0 1 1 1 1
  spline S51 degree 2 poles (233.0002, -100.9949) (230.4484, -100.8907) (229.9999, -99.995) knots 0 0 0 1 1 1
  spline S52 degree 2 poles (229.9999, -99.995) (228.7609, -97.5733) (229.9999, -94.9948) knots 0 0 0 1 1 1
  spline S53 degree 2 poles (229.9999, -94.9948) (225.0439, -92.9391) (225.0002, -89.9945) knots 0 0 0 1 1 1
  spline S54 degree 3 poles (225.0002, -89.9945) (225.0477, -78.8539) (225.2253, -67.7119) (225.0002, -56.5723) knots 0 0 0 0 1 1 1 1
  line L104 (225.0002, -56.5723) -> (217.904, -56.5723)
  line L105 (217.904, -56.5723) -> (217.0002, -207.9946)
  spline S55 degree 2 poles (217.0002, -207.9946) (217.04, -209.9459) (214.9998, -209.9945) knots 0 0 0 1 1 1
  line L106 (214.9998, -209.9945) -> (171.9998, -209.9919)
  spline S56 degree 2 poles (171.9998, -209.9919) (169.9601, -210.0255) (169.9999, -207.9946) knots 0 0 0 1 1 1
  line L107 (169.9999, -207.9946) -> (169.9456, -61.9947)
  line L108 (169.9456, -61.9947) -> (162.9455, -61.9947)
  line L109 (162.9455, -61.9947) -> (162.9998, -105.9946)
  line L110 (162.9998, -105.9946) -> (158.0002, -105.9946)
  line L111 (158.0002, -105.9946) -> (158.0002, -109.9948)
  line L112 (158.0002, -109.9948) -> (152.9999, -109.9948)
  line L113 (152.9999, -109.9948) -> (152.9999, -106.2116)
  line L114 (152.9999, -106.2116) -> (147.0783, -106.2116)
  line L115 (147.0783, -106.2116) -> (146.9997, -152.9948)
  line L116 (146.9997, -152.9948) -> (137.9998, -152.9948)
  line L117 (137.9998, -152.9948) -> (137.9998, -147.9946)
  line L118 (137.9998, -147.9946) -> (125.0001, -147.9946)
  line L119 (125.0001, -147.9946) -> (125.0001, -159.9949)
  line L120 (125.0001, -159.9949) -> (112.9998, -159.9949)
  line L121 (112.9998, -159.9949) -> (112.9135, -43.9948)
  line L122 (112.9135, -43.9948) -> (106.0003, -43.9948)
  line L123 (106.0003, -43.9948) -> (106.0003, -54.9946)
  line L124 (106.0003, -54.9946) -> (102, -54.9946)
  line L125 (102, -54.9946) -> (102, -75.9949)
  line L126 (102, -75.9949) -> (102, -81.995)
  line L127 (102, -81.995) -> (99.0002, -99.995)
  line L128 (99.0002, -99.995) -> (95.9998, -81.995)
  line L129 (95.9998, -81.995) -> (95.9998, -76.0739)
  line L130 (95.9998, -76.0739) -> (89.9666, -76.0739)
  line L131 (89.9666, -76.0739) -> (90.0002, -81.995)
  line L132 (90.0002, -81.995) -> (87.9998, -81.995)
  line L133 (87.9998, -81.995) -> (87.9998, -84.9948)
  line L134 (87.9998, -84.9948) -> (85.9999, -84.9948)
  line L135 (85.9999, -84.9948) -> (85.9999, -87.9947)
  line L136 (85.9999, -87.9947) -> (84, -87.9947)
  line L137 (84, -87.9947) -> (84, -90.995)
  line L138 (84, -90.995) -> (82.0002, -90.995)
  line L139 (82.0002, -90.995) -> (82.0002, -93.9948)
  line L140 (82.0002, -93.9948) -> (79.9998, -93.9948)
  line L141 (79.9998, -93.9948) -> (79.9998, -96.9946)
  line L142 (79.9998, -96.9946) -> (77.9999, -96.9946)
  line L143 (77.9999, -96.9946) -> (77.9999, -99.995)
  line L144 (77.9999, -99.995) -> (76, -99.995)
  line L145 (76, -99.995) -> (76, -102.9948)
  line L146 (76, -102.9948) -> (74.0001, -102.9948)
  line L147 (74.0001, -102.9948) -> (70.9998, -135.9948)
  line L148 (70.9998, -135.9948) -> (69.9999, -135.9948)
  line L149 (69.9999, -135.9948) -> (67, -102.9948)
  line L150 (67, -102.9948) -> (65.0002, -102.9948)
  line L151 (65.0002, -102.9948) -> (65.0503, -99.995)
  line L152 (65.0503, -99.995) -> (62.9998, -99.995)
  line L153 (62.9998, -99.995) -> (62.9998, -96.9946)
  line L154 (62.9998, -96.9946) -> (60.9999, -96.9946)
  line L155 (60.9999, -96.9946) -> (60.9999, -93.9948)
  line L156 (60.9999, -93.9948) -> (59, -93.9948)
  line L157 (59, -93.9948) -> (59, -90.995)
  line L158 (59, -90.995) -> (57.0001, -90.995)
  line L159 (57.0001, -90.995) -> (57.0001, -87.9947)
  line L160 (57.0001, -87.9947) -> (54.9997, -87.9947)
  line L161 (54.9997, -87.9947) -> (54.9997, -84.9948)
  line L162 (54.9997, -84.9948) -> (52.9999, -84.9948)
  line L163 (52.9999, -84.9948) -> (52.9999, -81.995)
  line L164 (52.9999, -81.995) -> (51, -81.995)
  line L165 (51, -81.995) -> (51, -75.9949)
  line L166 (51, -75.9949) -> (44.9998, -75.9949)
  line L167 (44.9998, -75.9949) -> (44.9998, -81.995)
  line L168 (44.9998, -81.995) -> (42, -99.995)
  line L169 (42, -99.995) -> (39.0002, -81.995)
  line L170 (39.0002, -81.995) -> (39.0002, -75.9949)
  line L171 (39.0002, -75.9949) -> (39.0002, -54.9946)
  line L172 (39.0002, -54.9946) -> (32.0001, -54.9946)
  line L173 (32.0001, -54.9946) -> (32.0022, -97.9946)
  line L174 (32.0022, -97.9946) -> (29.5047, -106.9945)
  line L175 (29.5047, -106.9945) -> (26.9999, -97.9946)
  line L176 (26.9999, -97.9946) -> (22.0002, -97.9946)
  line L177 (22.0002, -97.9946) -> (22.0002, -116.995)
  line L178 (22.0002, -116.995) -> (23.0002, -120.9947)
  line L179 (23.0002, -120.9947) -> (16.0001, -142.9949)
  line L180 (16.0001, -142.9949) -> (9, -120.9947)
  line L181 (9, -120.9947) -> (9.9999, -116.995)
  line L182 (9.9999, -116.995) -> (9.9999, -97.9946)
  line L183 (9.9999, -97.9946) -> (5.0002, -97.9946)
  line L184 (5.0002, -97.9946) -> (2.5068, -106.9945)
  line L185 (2.5068, -106.9945) -> (0, -97.9946)
  line L186 (0, -97.9946) -> (0, 0.0052)
  line L187 (0, 0.0052) -> (690, 0.0052)
  line L188 (690, 0.0052) -> (690, -39.9948)
  line L189 (690, -39.9948) -> (670.3637, -39.995)
  line L190 (670.3637, -39.995) -> (670.3637, -47.2783)
  spline S57 degree 3 poles (670.3637, -47.2783) (680, -47.9948) (687, -54.9948) (690, -61.9948) knots 0 0 0 0 1 1 1 1
  line L191 (690, -61.9948) -> (690, -84.9948)
  line L192 (690, -84.9948) -> (655, -84.9948)
  line L193 (655, -84.9948) -> (655, -89.9948)
  line L194 (655, -89.9948) -> (636, -89.9948)
  line L195 (636, -89.9948) -> (635, -121.9948)
  line L196 (635, -121.9948) -> (641, -121.9948)
  line L197 (641, -121.9948) -> (641, -123.9948)
  spline S58 degree 2 poles (641, -123.9948) (639, -124.0048) (639, -126.9948) knots 0 0 0 1 1 1
  spline S59 degree 2 poles (639, -126.9948) (639, -130.0299) (641, -130.0299) knots 0 0 0 1 1 1
  line L198 (641, -130.0299) -> (641, -131.9948)
  spline S60 degree 2 poles (641, -131.9948) (639, -132.0137) (639, -134.9948) knots 0 0 0 1 1 1
  spline S61 degree 2 poles (639, -134.9948) (639, -137.9948) (641, -137.9948) knots 0 0 0 1 1 1
  line L199 (641, -137.9948) -> (641, -139.9948)
  line L200 (641, -139.9948) -> (635, -139.9948)
  line L201 (635, -139.9948) -> (635, -145.9948)
  line L202 (635, -145.9948) -> (641, -147.9948)
  line L203 (641, -147.9948) -> (641, -157.9948)
  line L204 (641, -157.9948) -> (635, -159.9948)
  line L205 (635, -159.9948) -> (635, -165.9948)
  line L206 (635, -165.9948) -> (637, -165.9948)
  spline S62 degree 3 poles (637, -165.9948) (637.975, -165.9948) (639.0932, -167.0197) (639.0932, -167.9948) knots 0 0 0 0 1 1 1 1
  spline S63 degree 3 poles (639.0932, -167.9948) (639.0932, -169.0367) (638.0932, -169.9948) (637.0932, -169.9948) knots 0 0 0 0 1 1 1 1
  line L207 (637.0932, -169.9948) -> (635, -169.9948)
  line L208 (635, -169.9948) -> (635, -174.9948)
  line L209 (635, -174.9948) -> (633, -184.9948)
  line L210 (633, -184.9948) -> (632, -204.9948)
  line L211 (632, -204.9948) -> (631, -226.9948)
  spline S64 degree 2 poles (631, -226.9948) (630, -233.7378) (629, -226.9948) knots 0 0 0 1 1 1
  line L212 (0, 0.0052) -> (138, 0.0052)
  line L213 (138, 0.0052) -> (138, 15.0052)
  line L214 (552, 0.0052) -> (690, 0.0052)
  line L215 (552, 15.0052) -> (552, 0.0052)
  line L216 (276, 0.0052) -> (414, 0.0052)
  line L217 (414, 0.0052) -> (414, 15.0052)
  line L218 (276, 15.0052) -> (276, 0.0052)
  line L219 (690, 15.0052) -> (690, 70.0052)
  line L220 (690, 70.0052) -> (0, 70.0052)
  line L221 (0, 70.0052) -> (0, 15.0052)
  line L222 (584, 15.0052) -> (584, 43.1302)
  line L223 (584, 43.1302) -> (569, 43.1302)
  line L224 (569, 43.1302) -> (569, 15.0052)
  line L225 (552, 15.0052) -> (569, 15.0052)
  line L226 (584, 15.0052) -> (690, 15.0052)
  line L227 (106, 15.0052) -> (106, 43.1302)
  line L228 (106, 43.1302) -> (121, 43.1302)
  line L229 (121, 43.1302) -> (121, 15.0052)
  line L230 (121, 15.0052) -> (138, 15.0052)
  line L231 (106, 15.0052) -> (0, 15.0052)
  line L232 (352.5, 15.0052) -> (352.5, 43.1302)
  line L233 (352.5, 43.1302) -> (337.5, 43.1302)
  line L234 (337.5, 43.1302) -> (337.5, 15.0052)
  line L235 (352.5, 15.0052) -> (414, 15.0052)
  line L236 (337.5, 15.0052) -> (276, 15.0052)
  dimension "d101" = 138
  dimension "d102" = 15
  dimension "d104" = 138
  dimension "d105" = 15
  dimension "d165" = 138
  dimension "d166" = 138
  dimension "d167" = 15
  dimension "d168" = 70
  dimension "d169" = 15
  dimension "d170" = 28.125
  dimension "d171" = 106
  dimension "d172" = 15
  dimension "d173" = 15
  dimension "d174" = 28.125
  dimension "d175" = 106
  dimension "d176" = 15
  dimension "d177" = 28.125
  dimension "d178" = 15
  dimension "d179" = 61.5
  dimension "d180" = 15
  constraint horizontal L212
  constraint vertical L213
  constraint collinear L187 L212
  constraint horizontal L214
  constraint vertical L215
  constraint coincident L187 L214.start
  constraint vertical L186.end L221.end
  constraint vertical L187.end L219.start
  constraint horizontal L216
  constraint vertical L217
  constraint vertical L218
  constraint coincident L187 L216.start
  constraint perpendicular L219 L220
  constraint vertical L222
  constraint horizontal L223
  constraint vertical L224
  constraint perpendicular L224 L225
  constraint perpendicular L219 L226
  constraint vertical L227
  constraint horizontal L228
  constraint vertical L229
  constraint perpendicular L213 L230
  constraint parallel L230 L231
  constraint vertical L232
  constraint horizontal L233
  constraint vertical L234
  constraint perpendicular L232 L235
  constraint perpendicular L218 L236
  measures "d101" distance of L213.end L221.end
  measures "d102" distance of L212.end L213.end
  measures "d104" distance of L219.start L215.start
  measures "d105" distance of L214.start L215.start
  measures "d165" distance of L217.end L218.start
  measures "d166" distance of L213 L218
  measures "d167" distance of L216.end L217.end
  measures "d168" distance of L187.end L219.end
  measures "d169" distance of L222.end L223.end
  measures "d170" distance of L224.end L223.end
  measures "d171" distance of L219 L222
  measures "d172" distance of L187 L226
  measures "d173" distance of L227.end L228.end
  measures "d174" distance of L227.start L227.end
  measures "d175" distance of L221 L227
  measures "d176" distance of L187 L231
  measures "d177" distance of L232.start L232.end
  measures "d178" distance of L232.end L233.end
  measures "d179" distance of L218.start L234
  measures "d180" distance of L187 L236